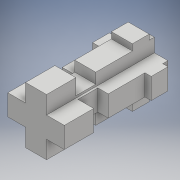
# Autodesk Inventor part: Empty
Saved by Autodesk Inventor 2018 (Build 220112000, 112)
## iProperties
Created: 2018-01-02
Part Number: Empty
Material: Generic
Document SubType Name: Modeling
Designer: suchanek
Density: 1 g/cm^3
Appearance: Default
Author: suchanek
Autodesk Inventor part; units mm, degrees
ref_plane "YZ Plane" through (0, 0, 0) normal (1, 0, 0) x (0, 1, 0)
ref_plane "XZ Plane" through (0, 0, 0) normal (0, 1, 0) x (-1, 0, 0)
ref_plane "XY Plane" through (0, 0, 0) normal (0, 0, 1) x (1, 0, 0)
sketch "Sketch1" plane through (0, 0, 0) normal (0, 0, 1) x (1, 0, 0)
  line L0 (0, 0) -> (-27, 0)
  line L1 (-27, 0) -> (27, 0)
  line L2 (27, 0) -> (27, 28)
  line L3 (27, 28) -> (-27, 28)
  line L4 (-27, 28) -> (-27, 0)
  line L5 (0, 28) -> (-12, 28)
  line L6 (-12, 28) -> (12, 28)
  line L7 (12, 28) -> (12, 47)
  line L8 (12, 47) -> (-12, 47)
  line L9 (-12, 47) -> (-12, 28)
  line L10 (0, 47) -> (-22, 47)
  line L11 (-22, 47) -> (22, 47)
  line L12 (22, 47) -> (22, 82)
  line L13 (22, 82) -> (-22, 82)
  line L14 (-22, 82) -> (-22, 47)
  line L15 (-22, 82) -> (-28, 82)
  line L16 (-28, 82) -> (28, 82)
  line L17 (28, 82) -> (28, 98)
  line L18 (28, 98) -> (-28, 98)
  line L19 (-28, 98) -> (-28, 82)
  line L20 (0, 98) -> (-23, 98)
  line L21 (-23, 98) -> (23, 98)
  line L22 (23, 98) -> (23, 103)
  line L23 (23, 103) -> (-23, 103)
  line L24 (-23, 103) -> (-23, 98)
  dimension "d0" = 27
  dimension "d1" = 54
  dimension "d2" = 28
  dimension "d3" = 12
  dimension "d4" = 24
  dimension "d5" = 19
  dimension "d6" = 22
  dimension "d7" = 44
  dimension "d8" = 35
  dimension "d9" = 6
  dimension "d10" = 56
  dimension "d11" = 16
  dimension "d12" = 23
  dimension "d13" = 46
  dimension "d14" = 5
  constraints: 50 end point, 10 parallel, 8 horizontal, 5 perpendicular, 3 midpoint, 2 point on line
  measures "d0" distance of L0.start L0.end
  measures "d1" distance of L3.end L2.end
  measures "d2" distance of L2.end L1.end
  measures "d3" distance of L5.start L5.end
  measures "d4" distance of L8.end L7.end
  measures "d5" distance of L7.end L6.end
  measures "d6" distance of L10.start L10.end
  measures "d7" distance of L13.end L12.end
  measures "d8" distance of L12.end L11.end
  measures "d9" distance of L13.end L15.end
  measures "d10" distance of L18.end L17.end
  measures "d11" distance of L17.end L16.end
  measures "d12" distance of L20.start L20.end
  measures "d13" distance of L23.end L22.end
  measures "d14" distance of L22.end L21.end
sketch "Sketch2" plane through (0, 0, 0) normal (1, 0, 0) x (0, 1, 0)
  line L0 (0, 0) -> (0, 27)
  line L1 (0, 27) -> (0, -27)
  line L2 (0, -27) -> (28, -27)
  line L3 (28, -27) -> (28, 27)
  line L4 (28, 27) -> (0, 27)
  line L5 (28, 0) -> (28, 12)
  line L6 (28, 12) -> (28, -12)
  line L7 (28, -12) -> (47, -12)
  line L8 (47, -12) -> (47, 12)
  line L9 (47, 12) -> (28, 12)
  line L10 (47, 0) -> (47, 22)
  line L11 (47, 22) -> (47, -22)
  line L12 (47, -22) -> (82, -22)
  line L13 (82, -22) -> (82, 22)
  line L14 (82, 22) -> (47, 22)
  line L15 (82, 22) -> (82, 28)
  line L16 (82, 28) -> (82, -28)
  line L17 (82, -28) -> (98, -28)
  line L18 (98, -28) -> (98, 28)
  line L19 (98, 28) -> (82, 28)
  line L20 (98, 0) -> (98, 23)
  line L21 (98, 23) -> (98, -23)
  line L22 (98, -23) -> (103, -23)
  line L23 (103, -23) -> (103, 23)
  line L24 (103, 23) -> (98, 23)
  point P0 (0, 0)
  dimension "d15" = 27
  dimension "d16" = 54
  dimension "d17" = 28
  dimension "d18" = 12
  dimension "d19" = 24
  dimension "d20" = 19
  dimension "d21" = 22
  dimension "d22" = 44
  dimension "d23" = 35
  dimension "d24" = 6
  dimension "d25" = 56
  dimension "d26" = 16
  dimension "d27" = 23
  dimension "d28" = 46
  dimension "d29" = 5
  constraints: 50 end point, 10 parallel, 5 perpendicular, 3 midpoint, 2 point on line
  measures "d15" distance of L0.start L0.end
  measures "d16" distance of L3.end L2.end
  measures "d17" distance of L2.end L1.end
  measures "d18" distance of L5.start L5.end
  measures "d19" distance of L8.end L7.end
  measures "d20" distance of L7.end L6.end
  measures "d21" distance of L10.start L10.end
  measures "d22" distance of L13.end L12.end
  measures "d23" distance of L12.end L11.end
  measures "d24" distance of L13.end L15.end
  measures "d25" distance of L18.end L17.end
  measures "d26" distance of L17.end L16.end
  measures "d27" distance of L20.start L20.end
  measures "d28" distance of L23.end L22.end
  measures "d29" distance of L22.end L21.end
extrude "Extrusion1" add sketch "Sketch1" along normal mid plane 20
extrude "Extrusion2" add sketch "Sketch2" along normal mid plane 20
body "Solid1"
